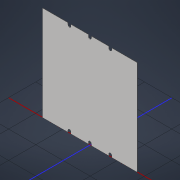
# Autodesk Inventor part: Heatbed Magnetic-Sheet
Saved by Autodesk Inventor 2022.2 (Build 262287010, 287A)
## iProperties
Created: 2022-03-13
Part Number: Heatbed Magnetic-Sheet
Material: Bronze, weiche Zinnbronze
Document SubType Name: Modeling
Designer: sleib
Density: 8.874 g/cm^3
Appearance: Bronze - satiniert
Author: sleib
Autodesk Inventor part; units mm, degrees
ref_plane "YZ Plane" through (0, 0, 0) normal (1, 0, 0) x (0, 1, 0)
ref_plane "XZ Plane" through (0, 0, 0) normal (0, 1, 0) x (-1, 0, 0)
ref_plane "XY Plane" through (0, 0, 0) normal (0, 0, 1) x (1, 0, 0)
sketch "Skizze1" plane through (0, 0, 0) normal (0, 0, 1) x (1, 0, 0)
  line L0 (175, -174) -> (174, -175) projected
  line L1 (175, -174) -> (175, 174) projected
  line L2 (174, 175) -> (175, 174) projected
  line L3 (174, 175) -> (80, 175) projected
  line L4 (80, 175) -> (80, 168) projected
  arc A0 (70, 168) -> (80, 168) centre (75, 168) ccw projected
  line L5 (70, 168) -> (70, 175) projected
  line L6 (70, 175) -> (5, 175) projected
  line L7 (5, 175) -> (5, 168) projected
  arc A1 (-5, 168) -> (5, 168) centre (0, 168) ccw projected
  line L8 (-5, 168) -> (-5, 175) projected
  line L9 (-5, 175) -> (-70, 175) projected
  line L10 (-70, 175) -> (-70, 168) projected
  arc A2 (-80, 168) -> (-70, 168) centre (-75, 168) ccw projected
  line L11 (-80, 168) -> (-80, 175) projected
  line L12 (-80, 175) -> (-174, 175) projected
  line L13 (-175, 174) -> (-174, 175) projected
  line L14 (-175, 174) -> (-175, -174) projected
  line L15 (-174, -175) -> (-175, -174) projected
  line L16 (-174, -175) -> (-80, -175) projected
  line L17 (-80, -175) -> (-80, -168) projected
  arc A3 (-70, -168) -> (-80, -168) centre (-75, -168) ccw projected
  line L18 (-70, -168) -> (-70, -175) projected
  line L19 (-70, -175) -> (-5, -175) projected
  line L20 (-5, -175) -> (-5, -168) projected
  arc A4 (5, -168) -> (-5, -168) centre (0, -168) ccw projected
  line L21 (5, -168) -> (5, -175) projected
  line L22 (5, -175) -> (70, -175) projected
  line L23 (70, -175) -> (70, -168) projected
  arc A5 (80, -168) -> (70, -168) centre (75, -168) ccw projected
  line L24 (80, -168) -> (80, -175) projected
  line L25 (80, -175) -> (174, -175) projected
  line L26 (174.5, 173.7929) -> (174.5, -173.7929)
  line L27 (174.5, -173.7929) -> (173.7929, -174.5)
  line L28 (173.7929, -174.5) -> (80.5, -174.5)
  line L29 (80.5, -174.5) -> (80.5, -168)
  arc A6 (80.5, -168) -> (69.5, -168) centre (75, -168) ccw
  line L30 (69.5, -168) -> (69.5, -174.5)
  line L31 (69.5, -174.5) -> (5.5, -174.5)
  line L32 (5.5, -174.5) -> (5.5, -168)
  arc A7 (5.5, -168) -> (-5.5, -168) centre (0, -168) ccw
  line L33 (-5.5, -168) -> (-5.5, -174.5)
  line L34 (-5.5, -174.5) -> (-69.5, -174.5)
  line L35 (-69.5, -174.5) -> (-69.5, -168)
  arc A8 (-69.5, -168) -> (-80.5, -168) centre (-75, -168) ccw
  line L36 (-80.5, -168) -> (-80.5, -174.5)
  line L37 (-80.5, -174.5) -> (-173.7929, -174.5)
  line L38 (-173.7929, -174.5) -> (-174.5, -173.7929)
  line L39 (-174.5, -173.7929) -> (-174.5, 173.7929)
  line L40 (-174.5, 173.7929) -> (-173.7929, 174.5)
  line L41 (-173.7929, 174.5) -> (-80.5, 174.5)
  line L42 (-80.5, 174.5) -> (-80.5, 168)
  arc A9 (-80.5, 168) -> (-69.5, 168) centre (-75, 168) ccw
  line L43 (-69.5, 168) -> (-69.5, 174.5)
  line L44 (-69.5, 174.5) -> (-5.5, 174.5)
  line L45 (-5.5, 174.5) -> (-5.5, 168)
  arc A10 (-5.5, 168) -> (5.5, 168) centre (0, 168) ccw
  line L46 (5.5, 168) -> (5.5, 174.5)
  line L47 (5.5, 174.5) -> (69.5, 174.5)
  line L48 (69.5, 174.5) -> (69.5, 168)
  arc A11 (69.5, 168) -> (80.5, 168) centre (75, 168) ccw
  line L49 (80.5, 168) -> (80.5, 174.5)
  line L50 (80.5, 174.5) -> (173.7929, 174.5)
  line L51 (173.7929, 174.5) -> (174.5, 173.7929)
  point P0 (0, 0)
  dimension "d0" = 0.5
  constraints: 52 end point, 12 point on circle, 6 centre point, 31 other
  measures "d0" distance between parallel lines of L1 L26
extrude "Extrusion1" add sketch "Skizze1" along normal blind 1 contours L26 L27 L28 L29 A6 L30 L31 L32 A7 L33 L34 L35 A8 L36 L37 L38 L39 L40 L41 L42 A9 L43 L44 L45 A10 L46 L47 L48 A11 L49 L50 L51
